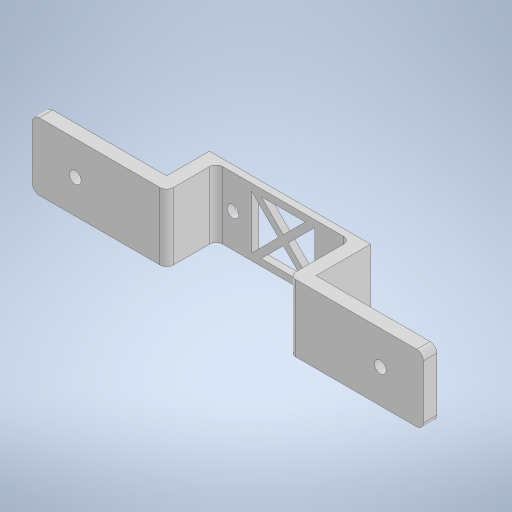
# Autodesk Inventor part: joint2_sup
Saved by Autodesk Inventor 2023 (Build 270158000, 158)
## iProperties
Created: 2023-04-29
Part Number: joint2_sup
Material: 一般
Document SubType Name: Modeling
Designer: taka2
Density: 1 g/cm^3
Appearance: 既定
Author: taka2
Autodesk Inventor part; units mm, degrees
ref_plane "YZ Plane" through (0, 0, 0) normal (1, 0, 0) x (0, 1, 0)
ref_plane "XZ Plane" through (0, 0, 0) normal (0, 1, 0) x (-1, 0, 0)
ref_plane "XY Plane" through (0, 0, 0) normal (0, 0, 1) x (1, 0, 0)
sketch "スケッチ1" plane through (0, 0, 0) normal (0, 1, 0) x (-1, 0, 0)
  line L0 (0, 20.7547) -> (0, -42.4528)
  line L1 (60, 16.75) -> (20, 16.75)
  line L2 (20, 16.75) -> (20, 2)
  line L3 (20, 2) -> (0, 2)
  line L4 (60, 16.75) -> (60, 12.75)
  line L5 (60, 12.75) -> (24, 12.75)
  line L6 (24, 12.75) -> (24, 0)
  line L7 (24, 0) -> (0, 0)
  line L8 (-20, 2) -> (0, 2)
  line L9 (-24, 0) -> (0, 0)
  line L10 (-24, 0) -> (-24, 16.25)
  line L11 (-24, 16.25) -> (-60, 16.25)
  line L12 (-60, 16.25) -> (-60, 20.25)
  line L13 (-60, 20.25) -> (-20, 20.25)
  line L14 (-20, 20.25) -> (-20, 2)
  dimension "d0" = 40
  dimension "d1" = 4
  dimension "d2" = 36
  dimension "d4" = 2
  dimension "d5" = 40
  dimension "d20" = 12.75
  dimension "d21" = 16.25
  dimension "d22" = 4
  dimension "d23" = 40
  dimension "d24" = 4
  constraints: 30 end point, 7 perpendicular, 5 point on line, 4 vertical, 2 horizontal, 2 symmetric about line
  measures "d0" distance of L1.start L1.end
  measures "d1" distance of L1.start L4.end
  measures "d2" distance of L4.end L5.end
  measures "d4" distance between parallel lines of L3 L7
  measures "d5" distance of L8.start L2.end
  measures "d20" distance of L5.end L6.end
  measures "d21" distance of L10.start L10.end
  measures "d22" distance of L11.end L12.end
  measures "d23" distance of L12.end L13.end
  measures "d24" distance between parallel lines of L14 L10
extrude "押し出し1" add sketch "スケッチ1" along normal blind 20
sketch "スケッチ2" plane through (24, 0, 0) normal (0, 0, -1) x (-1, 0, 0)
  line L0 (0, 10) -> (48, 10)
  line L1 (48, 0) -> (48, 20) projected
  line L2 (24, 0) -> (24, 20)
  line L3 (0, 20) -> (48, 20) projected
  circle A0 centre (9, 10) radius 1.75
  line L4 (14.5858, 18) -> (14.5858, 2)
  line L5 (14.5858, 2) -> (30.5858, 2)
  line L6 (30.5858, 2) -> (14.5858, 18)
  circle A1 centre (39, 10) radius 1.75
  line L7 (33.4142, 18) -> (33.4142, 2)
  line L8 (33.4142, 18) -> (17.4142, 18)
  line L9 (17.4142, 18) -> (33.4142, 2)
  line L10 (33.4142, 18) -> (17.4142, 2)
  line L11 (14.5858, 2) -> (30.5858, 18)
  point P0 (25.4142, 10)
  point P1 (24, 8.5858)
  point P2 (22.5858, 10)
  point P3 (24, 11.4142)
  dimension "d8" = 16
  dimension "d9" = 3.5
  dimension "d11" = 30
  dimension "d19" = 2
  dimension "d27" = 2
  constraints: 20 end point, 4 symmetric about line, 3 point on line, 2 centre point, 2 equal length, 2 midpoint, 2 vertical, 1 horizontal, 1 parallel, 1 perpendicular, 1 other
  measures "d8" distance of L4.start L4.end
  measures "d9" diameter of A0
  measures "d11" distance of A1.centre A0.centre
  measures "d19" distance between parallel lines of L9 L6
  measures "d27" distance between parallel lines of L10 L11
extrude "押し出し2" cut sketch "スケッチ2" against normal through all contours A1 L0 | L0 A1 | A0 L0 | L0 A0 | L7 L9 L0 | L0 L10 L7 | L8 L11 L2 | L2 L9 L8 | L6 L5 L2 | L2 L5 L10 | L11 L4 L0 | L0 L4 L6
sketch "スケッチ3" plane through (20, 0, 16.25) normal (0, 0, 1) x (1, 0, 0)
  line L0 (-80, 0) -> (-80, 20) projected
  line L1 (-80, 10) -> (40, 10)
  circle A0 centre (27.1661, 10) radius 1.75
  circle A1 centre (-67.25, 10) radius 1.75
  line L2 (40, 0) -> (40, 20) projected
  point P0 (-20, 0)
  dimension "d14" = 3.5
  dimension "d16" = 12.75
  constraints: 2 centre point, 2 end point, 2 midpoint, 2 point on line, 1 equal radius
  measures "d14" diameter of A0
  measures "d16" distance from line of L0 A1.centre
extrude "押し出し3" cut sketch "スケッチ3" along normal through all both and the other way through all
fillet "フィレット1" radius 2 4 edges at (60, 20, 18.25) (60, 0, 18.25) (-60, 20, 14.75) (-60, 0, 14.75)
fillet "フィレット2" radius 2 4 edges at (-20, 10, 16.75) (-20, 10, 2) (20, 10, 2) (20, 10, 20.25)
